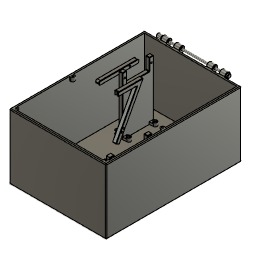
Useless_box (Autodesk Fusion 360 design; units mm, degrees)
Autodesk Fusion 360 part; units mm, degrees
note: some values were not read from the file. Set by a fixed rule: which face or edge a step refers to.
(part 1 of 2)
sketch "Sketch1" plane through (0, 0, 0) normal (0, 1, 0) x (1, 0, 0) in component "Box"
  line L0 (-60, -85) -> (60, -85)
  line L1 (60, -85) -> (60, 85)
  line L2 (60, 85) -> (-60, 85)
  line L3 (-60, 85) -> (-60, -85)
  line L4 (-60, -85) -> (60, 85) construction
  line L5 (60, -85) -> (-60, 85) construction
  dimension "d20" = 120
  dimension "d21" = 170
  constraint horizontal L0
  constraint perpendicular L0 L1
  constraint parallel L0 L2
  constraint parallel L1 L3
  constraint coincident L4 origin
  constraint coincident L5 origin
  measures "d20" distance of L1.end L2.end
  measures "d21" distance of L0.end L1.end
extrude "Extrude1" add sketch "Sketch1" along normal blind 3 makes body 1 in component "Box"
move_body "Move1" bodies 1 to x (1, 0, 0) y (0, 1, 0) z (0, 0, 1) at (0, 0, -10) in component "Box"
sketch "Sketch2" plane through (0, 3, 0) normal (0, 1, 0) x (-1, 0, 0) in component "Box"
  line L0 (60, -95) -> (60, 75)
  line L1 (60, 75) -> (-60, 75)
  line L2 (-60, 75) -> (-60, -95)
  line L3 (-60, -95) -> (60, -95)
  line L4 (60, -95) -> (60, -98)
  line L5 (60, -98) -> (63, -98)
  line L6 (63, -98) -> (63, 78)
  line L7 (63, 78) -> (-63, 78)
  line L8 (-63, 78) -> (-63, -98)
  line L9 (-63, -98) -> (63, -98)
  dimension "d26" = 3
  dimension "d27" = 3
  dimension "d28" = 176
  dimension "d29" = 126
  dimension "d30" = 176
  dimension "d31" = 126
  constraint coincident L0.start L3.end
  constraint perpendicular L3 L4
  constraint perpendicular L4 L5
  constraint perpendicular L5 L6
  constraint perpendicular L6 L7
  constraint perpendicular L7 L8
  constraint perpendicular L8 L9
  measures "d26" distance of L0.start L4.end
  measures "d27" distance of L4.end L5.end
  measures "d28" distance of L5.end L6.end
  measures "d29" distance of L6.end L7.end
  measures "d30" distance of L7.end L8.end
  measures "d31" distance of L8.end L5.end
extrude "Extrude2" add sketch "Sketch2" against normal up to surface (3 mm away) bodies 1 in component "Box"
sketch "Sketch3" plane through (0, 3, 0) normal (0, 1, 0) x (-1, 0, 0) in component "Box"
  line L0 (-63, -98) -> (63, -98)
  line L1 (63, -98) -> (63, 78)
  line L2 (63, 78) -> (-63, 78)
  line L3 (-63, 78) -> (-63, -98)
  line L4 (-60, -95) -> (60, -95)
  line L5 (60, -95) -> (60, 75)
  line L6 (60, 75) -> (-60, 75)
  line L7 (-60, 75) -> (-60, -95)
  line L8 (-60, -95) -> (60, 75) construction
  line L9 (60, -95) -> (-60, 75) construction
  line L10 (-14, -85) -> (-50, -85)
  line L11 (-50, -85) -> (-50, -29)
  line L12 (-50, -29) -> (-14, -29)
  line L13 (-14, -29) -> (-14, -85)
  circle A0 centre (-14, -85) radius 2.5
  circle A1 centre (-50, -85) radius 2.5
  circle A2 centre (-50, -29) radius 2.5
  circle A3 centre (-14, -29) radius 2.5
  circle A4 centre (-14, -85) radius 1.05
  circle A5 centre (-50, -85) radius 1.05
  circle A6 centre (-50, -29) radius 1.05
  circle A7 centre (-14, -29) radius 1.05
  line L14 (0, 0) -> (-22, 0)
  line L15 (-22, 0) -> (-22, -18)
  line L16 (-22, -18) -> (-27, -18)
  line L17 (-27, -18) -> (-27, 37)
  line L18 (-27, 37) -> (-22, 37)
  line L19 (-22, 37) -> (-22, 0)
  line L20 (39, -78) -> (34, -78)
  line L21 (39, -78) -> (39, -43.5)
  line L22 (34, -78) -> (34, -43.5)
  line L23 (34, -43.5) -> (39, -43.5)
  line L24 (39, -78) -> (39, -81)
  line L25 (39, -81) -> (34, -81)
  line L26 (34, -81) -> (34, -78)
  line L27 (39, -43.5) -> (39, -40.5)
  line L28 (39, -40.5) -> (34, -40.5)
  line L29 (34, -40.5) -> (34, -43.5)
  point P0 (0, -10)
  dimension "d34" = 120
  dimension "d35" = 170
  dimension "d36" = 36
  dimension "d37" = 56
  dimension "d38" = 10
  dimension "d39" = 10
  dimension "d40" = 5
  dimension "d41" = 5
  dimension "d42" = 5
  dimension "d43" = 5
  dimension "d44" = 2.1
  dimension "d45" = 2.1
  dimension "d46" = 2.1
  dimension "d47" = 2.1
  dimension "d50" = 22
  dimension "d51" = 18
  dimension "d52" = 5
  dimension "d53" = 55
  dimension "d54" = 5
  dimension "d76" = 5
  dimension "d77" = 17
  dimension "d78" = 34.5
  dimension "d79" = 21
  dimension "d80" = 3
  dimension "d81" = 5
  dimension "d82" = 3
  dimension "d83" = 5
  constraint horizontal L4
  constraint perpendicular L4 L5
  constraint parallel L4 L6
  constraint parallel L5 L7
  constraint coincident L8 P0
  constraint coincident L9 P0
  constraint horizontal L10
  constraint vertical L11
  constraint horizontal L12
  constraint vertical L13
  constraint coincident L10.start L13.end
  constraint coincident L10.end L11.start
  constraint coincident L11.end L12.start
  constraint coincident L12.end L13.start
  constraint concentric A0 A4
  constraint concentric A1 A5
  constraint concentric A2 A6
  constraint concentric A3 A7
  constraint coincident L14.start origin
  constraint horizontal L14
  constraint perpendicular L14 L15
  constraint perpendicular L15 L16
  constraint perpendicular L16 L17
  constraint perpendicular L17 L18
  constraint perpendicular L5 L20
  constraint perpendicular L20 L21
  constraint perpendicular L20 L22
  constraint perpendicular L21 L23
  constraint perpendicular L20 L24
  constraint perpendicular L24 L25
  constraint perpendicular L23 L27
  constraint perpendicular L27 L28
  measures "d34" distance of L5.end L6.end
  measures "d35" distance of L4.end L5.end
  measures "d36" distance of L10.start L10.end
  measures "d37" distance of L10.start L12.end
  measures "d38" distance of L7 L11
  measures "d39" distance of L4 L10
  measures "d40" diameter of A0
  measures "d41" diameter of A1
  measures "d42" diameter of A2
  measures "d43" diameter of A3
  measures "d44" diameter of A4
  measures "d45" diameter of A5
  measures "d46" diameter of A6
  measures "d47" diameter of A7
  measures "d50" distance of L14.start L14.end
  measures "d51" distance of L14.end L15.end
  measures "d52" distance of L15.end L16.end
  measures "d53" distance of L16.end L17.end
  measures "d54" distance of L17.end L18.end
  measures "d76" distance of L20.start L20.end
  measures "d77" distance of L4 L20
  measures "d78" distance of L20.start L21.end
  measures "d79" distance of L5 L21
  measures "d80" distance of L20.start L24.end
  measures "d81" distance of L24.end L25.end
  measures "d82" distance of L21.end L27.end
  measures "d83" distance of L27.end L28.end
extrude "Extrude9" add sketch "Sketch3" along normal blind 12 contours L10 L11 A1 A5 | L10 L11 A1 A5 | L10 L13 A0 A4 | L10 L13 A0 A4 | L11 L12 A2 A6 | L11 L12 A2 A6 | L12 L13 A3 A7 | L12 L13 A3 A7 bodies 1 in component "Box"
sketch "Sketch1 (2)" plane through (0, 3, 0) normal (0, 1, 0) x (-1, 0, 0) in component "Switch_servo_mount"
  circle A0 centre (-50, -29) radius 2.5
  circle A1 centre (-14, -29) radius 2.5
  line L0 (-63, -98) -> (63, -98)
  line L1 (63, -98) -> (63, 78)
  line L2 (63, 78) -> (-63, 78)
  line L3 (-63, 78) -> (-63, -98)
  circle A2 centre (-14, -85) radius 2.5
  circle A3 centre (-50, -85) radius 2.5
  line L4 (-22, -18) -> (-27, -18)
  line L5 (-27, -18) -> (-27, 37)
  line L6 (-27, 37) -> (-22, 37)
  line L7 (-22, 37) -> (-22, -18)
  line L8 (0, 0) -> (-22, 0) construction
  line L9 (-22, -18) -> (-17, -18)
  circle A4 centre (-17, -15) radius 2.5
  circle A5 centre (-32, -15) radius 2.5
  line L10 (-22, -18) -> (-27, -18)
  circle A6 centre (-17, 34) radius 2.5
  circle A7 centre (-32, 34) radius 2.5
  line L11 (-27, 37) -> (-22, 37)
  line L12 (-22, 37) -> (-16.7571, 36.4882)
  line L13 (-27, 37) -> (-32.2429, 36.4882)
  line L14 (-32.2429, 31.5118) -> (-27, 31)
  line L15 (-17, 31.5) -> (-22, 31)
  line L16 (-22, -18) -> (-16.7571, -17.4882)
  line L17 (-16.7571, -12.5118) -> (-22, -12)
  line L18 (-27, -18) -> (-32.2429, -17.4882)
  line L19 (-32, -12.5) -> (-27, -11.7993)
  circle A8 centre (-17, -15) radius 1.05
  circle A9 centre (-32, -15) radius 1.05
  circle A10 centre (-17, 34) radius 1.05
  circle A11 centre (-32, 34) radius 1.05
  line L20 (39, -40.5) -> (39, -81)
  line L21 (39, -81) -> (34, -81)
  line L22 (34, -81) -> (34, -40.5)
  line L23 (34, -40.5) -> (39, -40.5)
  circle A12 centre (44, -78) radius 2.5
  circle A13 centre (29, -78) radius 2.5
  circle A14 centre (44, -43.5) radius 2.5
  circle A15 centre (29, -43.5) radius 2.5
  line L24 (39, -40.5) -> (34, -40.5)
  line L25 (34, -81) -> (28.7571, -80.4882)
  line L26 (39, -81) -> (44.2429, -80.4882)
  line L27 (44, -75.5) -> (39, -75.0119)
  line L28 (29, -75.5) -> (34, -75.0119)
  line L29 (39, -40.5) -> (44.2429, -41.0118)
  line L30 (34, -40.5) -> (28.7571, -41.0118)
  line L31 (28.7571, -45.9882) -> (34, -46.5)
  line L32 (39, -46.5) -> (44.2429, -45.9882)
  point P0 (34, -78)
  point P1 (39, -78)
  point P2 (39, -43.5)
  point P3 (34, -43.5)
  dimension "d118" = 5
  dimension "d119" = 5
  dimension "d120" = 5
  dimension "d121" = 3
  dimension "d122" = 5
  dimension "d123" = 3
  dimension "d124" = 5
  dimension "d125" = 5
  dimension "d126" = 5
  dimension "d127" = 3
  dimension "d128" = 3
  dimension "d129" = 5
  dimension "d130" = 5
  dimension "d131" = 2.1
  dimension "d132" = 2.1
  dimension "d133" = 2.1
  dimension "d134" = 2.1
  dimension "d193" = 5
  dimension "d196" = 5
  dimension "d197" = 5
  dimension "d198" = 5
  dimension "d199" = 5
  dimension "d200" = 5
  dimension "d201" = 5
  dimension "d202" = 5
  dimension "d203" = 5
  dimension "d204" = 3
  dimension "d205" = 3
  dimension "d206" = 3
  dimension "d207" = 3
  constraint horizontal L4
  constraint perpendicular L4 L5
  constraint perpendicular L5 L6
  constraint perpendicular L4 L7
  constraint coincident L8.start origin
  constraint coincident L7 L8.end
  constraint perpendicular L7 L8
  constraint perpendicular L7 L9
  constraint coincident L6.end L7.start
  constraint coincident A6 L12.end
  constraint tangent A6 L12
  constraint coincident L5.end L6.start
  constraint coincident A7 L13.end
  constraint tangent A7 L13
  constraint coincident A7 L14.start
  constraint coincident L5 L14.end
  constraint tangent A7 L14
  constraint coincident A6 L15.start
  constraint coincident L7 L15.end
  constraint coincident L4.start L7.end
  constraint coincident A4 L16.end
  constraint tangent A4 L16
  constraint coincident A4 L17.start
  constraint coincident L7 L17.end
  constraint tangent A4 L17
  constraint coincident L4.end L5.start
  constraint coincident A5 L18.end
  constraint tangent A5 L18
  constraint coincident A5 L19.start
  constraint coincident L5 L19.end
  constraint concentric A4 A8
  constraint concentric A5 A9
  constraint concentric A6 A10
  constraint concentric A7 A11
  constraint vertical L20
  constraint perpendicular L20 L21
  constraint perpendicular L21 L22
  constraint perpendicular L20 L23
  constraint coincident A13 L25.end
  constraint tangent A13 L25
  constraint coincident A12 L26.end
  constraint tangent A12 L26
  constraint coincident A12 L27.start
  constraint coincident L20 L27.end
  constraint parallel L25 L27
  constraint coincident A13 L28.start
  constraint coincident L22 L28.end
  constraint parallel L26 L28
  constraint coincident A14 L29.end
  constraint tangent A14 L29
  constraint coincident L22.end L23.start
  constraint coincident A15 L30.end
  constraint tangent A15 L30
  constraint coincident A15 L31.start
  constraint coincident L22 L31.end
  constraint tangent A15 L31
  constraint coincident L20 L32.start
  constraint coincident A14 L32.end
  constraint tangent A14 L32
  measures "d118" distance of L4.start L9.end
  measures "d119" diameter of A4
  measures "d120" diameter of A5
  measures "d121" distance of L9 A4.centre
  measures "d122" distance of L7 A4.centre
  measures "d123" distance of A5.centre L10
  measures "d124" distance of L5 A5.centre
  measures "d125" diameter of A6
  measures "d126" diameter of A7
  measures "d127" distance of A7.centre L11
  measures "d128" distance of L6 A6.centre
  measures "d129" distance of L7 A6.centre
  measures "d130" distance of L5 A7.centre
  measures "d131" diameter of A8
  measures "d132" diameter of A9
  measures "d133" diameter of A10
  measures "d134" diameter of A11
  measures "d193" distance of L20.end L21.end
  measures "d196" diameter of A12
  measures "d197" diameter of A13
  measures "d198" diameter of A14
  measures "d199" diameter of A15
  measures "d200" distance of A13.centre P0
  measures "d201" distance of A12.centre P1
  measures "d202" distance of A14.centre P2
  measures "d203" horizontal distance of A15.centre P3
  measures "d204" distance of L23 A15.centre
  measures "d205" distance of A14.centre L24
  measures "d206" distance of L21 A12.centre
  measures "d207" distance of L21 A13.centre
sketch "Sketch1 (3)" plane through (0, 3, 0) normal (0, 1, 0) x (-1, 0, 0) in component "Lid_servo_mount"
  circle A0 centre (-50, -29) radius 2.5
  circle A1 centre (-14, -29) radius 2.5
  line L0 (-63, -98) -> (63, -98)
  line L1 (63, -98) -> (63, 78)
  line L2 (63, 78) -> (-63, 78)
  line L3 (-63, 78) -> (-63, -98)
  circle A2 centre (-14, -85) radius 2.5
  circle A3 centre (-50, -85) radius 2.5
  line L4 (34, -40.5) -> (39, -40.5)
  line L5 (39, -40.5) -> (39, -81)
  line L6 (39, -81) -> (34, -81)
  line L7 (34, -81) -> (34, -40.5)
  circle A4 centre (44, -78) radius 2.5
  circle A5 centre (29, -78) radius 2.5
  circle A6 centre (44, -43.5) radius 2.5
  circle A7 centre (29, -43.5) radius 2.5
  line L8 (39, -40.5) -> (44.2429, -41.0118)
  line L9 (44.2429, -45.9882) -> (39, -46.5)
  line L10 (34, -40.5) -> (28.7571, -41.0118)
  line L11 (28.7571, -45.9882) -> (34, -46.5)
  line L12 (39, -81) -> (44.2429, -80.4882)
  line L13 (34, -81) -> (28.7571, -80.4882)
  line L14 (28.7571, -75.5118) -> (34, -75)
  line L15 (39, -75) -> (44.2429, -75.5118)
  circle A8 centre (44, -78) radius 1.05
  circle A9 centre (29, -78) radius 1.05
  circle A10 centre (29, -43.5) radius 1.05
  circle A11 centre (44, -43.5) radius 1.05
  dimension "d208" = 5
  dimension "d209" = 5
  dimension "d210" = 5
  dimension "d211" = 5
  dimension "d212" = 5
  dimension "d213" = 5
  dimension "d214" = 2.1
  dimension "d215" = 2.1
  dimension "d216" = 2.1
  dimension "d217" = 2.1
  constraint horizontal L4
  constraint perpendicular L4 L5
  constraint perpendicular L5 L6
  constraint coincident A6 L8.end
  constraint tangent A6 L8
  constraint coincident A6 L9.start
  constraint coincident L5 L9.end
  constraint tangent A6 L9
  constraint coincident A7 L10.end
  constraint tangent A7 L10
  constraint coincident A7 L11.start
  constraint coincident L7 L11.end
  constraint tangent A7 L11
  constraint coincident A4 L12.end
  constraint tangent A4 L12
  constraint coincident A5 L13.end
  constraint tangent A5 L13
  constraint coincident A5 L14.start
  constraint coincident L7 L14.end
  constraint tangent A5 L14
  constraint coincident L5 L15.start
  constraint coincident A4 L15.end
  constraint tangent A4 L15
  constraint concentric A4 A8
  constraint concentric A5 A9
  constraint concentric A7 A10
  constraint concentric A6 A11
  measures "d208" distance of L4.start L4.end
  measures "d209" distance of L5.end L6.end
  measures "d210" diameter of A4
  measures "d211" diameter of A5
  measures "d212" diameter of A6
  measures "d213" diameter of A7
  measures "d214" diameter of A8
  measures "d215" diameter of A9
  measures "d216" diameter of A10
  measures "d217" diameter of A11
extrude "Extrude1'" add sketch "Sketch1 (3)" along normal blind 3 separate body contours L5 A6 L8 L9 makes body 2 in component "Lid_servo_mount"
extrude "Extrude2'" add sketch "Sketch1 (2)" along normal blind 75 contours L20 L21 L22 L23 L24 bodies 2 in component "Lid_servo_mount"
extrude "Extrude3" add sketch "Sketch1 (2)" along normal blind 3 contours L22 A15 L30 L31 | L20 A12 L26 L27 | L22 A13 L25 L28 bodies 2 in component "Lid_servo_mount"
extrude "Extrude4" add sketch "Sketch1 (3)" along normal blind 5 contours A7 | A6 | A5 | A4 bodies 2 in component "Lid_servo_mount"
extrude "Extrude1''" add sketch "Sketch1 (2)" along normal blind 49 separate body contours L4 L5 L6 L7 L10 L11 makes body 3 in component "Switch_servo_mount"
extrude "Extrude2''" add sketch "Sketch1 (2)" along normal blind 3 contours L7 A4 L16 L17 | L5 A5 L18 L19 | L7 A6 L12 L15 | L5 A7 L13 L14 bodies 3 in component "Switch_servo_mount"
extrude "Extrude3'" add sketch "Sketch1 (2)" along normal blind 5 contours A4 | A5 | A6 | A7 bodies 3 in component "Switch_servo_mount"
sketch "Sketch2 (2)" plane through (22, 0, 0) normal (-1, 0, 0) x (0, 0, 1) in component "Switch_servo_mount"
  line L0 (-12, 6) -> (-12, 3)
  line L1 (-12, 3) -> (31, 3)
  line L2 (31, 3) -> (31, 6)
  line L3 (31, 6) -> (37, 6)
  line L4 (37, 6) -> (37, 52)
  line L5 (37, 52) -> (-18, 52)
  line L6 (-18, 52) -> (-18, 6)
  line L7 (-18, 6) -> (-12, 6)
  line L8 (-15, 52) -> (-15, 32) construction
  line L9 (34, 52) -> (34, 32) construction
  line L10 (31, 52) -> (31, 32) construction
  line L11 (-12, 52) -> (-12, 32) construction
  circle A0 centre (-15, 45) radius 0.85
  circle A1 centre (-15, 39) radius 0.85
  circle A2 centre (34, 45) radius 0.85
  line L12 (-15, 42) -> (34, 42) construction
  circle A3 centre (34, 39) radius 0.85
  line L13 (-12, 32) -> (31, 32)
  line L14 (31, 52) -> (31, 32)
  line L15 (31, 52) -> (-12, 52)
  line L16 (-12, 52) -> (-12, 32)
  circle A4 centre (0, 42) radius 2.5
  dimension "d141" = 20
  dimension "d142" = 20
  dimension "d143" = 3
  dimension "d144" = 3
  dimension "d145" = 20
  dimension "d147" = 20
  dimension "d148" = 3
  dimension "d149" = 3
  dimension "d150" = 1.7
  dimension "d151" = 1.7
  dimension "d152" = 1.7
  dimension "d153" = 1.7
  dimension "d154" = 3
  dimension "d155" = 3
  dimension "d156" = 3
  dimension "d157" = 3
  dimension "d158" = 5
  dimension "d159" = 10
  dimension "d161" = 15
  constraint coincident L5 L8.start
  constraint perpendicular L5 L8
  constraint coincident L5 L9.start
  constraint perpendicular L5 L9
  constraint coincident L5 L10.start
  constraint perpendicular L5 L10
  constraint coincident L5 L11.start
  constraint perpendicular L5 L11
  constraint coincident L8 A0.centre
  constraint coincident L8 A1.centre
  constraint coincident L9 A2.centre
  constraint midpoint L8 L12.start
  constraint midpoint L9 L12.end
  constraint coincident L9 A3.centre
  measures "d141" distance of L8.start L8.end
  measures "d142" distance of L9.start L9.end
  measures "d143" distance of L6 L8
  measures "d144" distance of L4 L9
  measures "d145" distance of L10.start L10.end
  measures "d147" distance of L11.start L11.end
  measures "d148" distance of L9 L10
  measures "d149" distance of L8 L11
  measures "d150" diameter of A0
  measures "d151" diameter of A1
  measures "d152" diameter of A2
  measures "d153" diameter of A3
  measures "d154" distance of A0.centre L12.start
  measures "d155" distance of A1.centre L12.start
  measures "d156" distance of L12.end A3.centre
  measures "d157" distance of A2.centre L12.end
  measures "d158" diameter of A4
  measures "d159" distance of L15 A4.centre
  measures "d161" distance of L12.start A4.centre
extrude "Extrude4'" cut sketch "Sketch2 (2)" against normal blind 5 contours L5 L13 L14 L15 L16 | A0 | A1 | A2 | A3 | A4 bodies 3 in component "Switch_servo_mount"
sketch "Sketch2 (3)" plane through (-39, 0, 0) normal (-1, 0, 0) x (0, 0, 1) in component "Lid_servo_mount"
  line L0 (-75.0119, 6) -> (-75.0119, 3)
  line L1 (-75.0119, 3) -> (-46.5, 3)
  line L2 (-46.5, 3) -> (-46.5, 6)
  line L3 (-46.5, 6) -> (-40.5, 6)
  line L4 (-40.5, 6) -> (-40.5, 78)
  line L5 (-40.5, 78) -> (-81, 78)
  line L6 (-81, 78) -> (-81, 6)
  line L7 (-81, 6) -> (-75.0119, 6)
  line L8 (-78, 78) -> (-78, 64.5) construction
  line L9 (-78, 64.5) -> (-43.5, 64.5)
  line L10 (-43.5, 64.5) -> (-40.5, 64.5)
  line L11 (-43.5, 64.5) -> (-43.5, 78) construction
  line L12 (-78, 71.25) -> (-43.5, 71.25) construction
  line L13 (-46, 78) -> (-46, 64.5)
  line L14 (-75.5, 78) -> (-75.5, 64.5)
  circle A0 centre (-78, 71.25) radius 1
  circle A1 centre (-43.5, 71.25) radius 1
  dimension "d226" = 13.5
  dimension "d227" = 3
  dimension "d228" = 34.5
  dimension "d229" = 3
  dimension "d230" = 2.5
  dimension "d231" = 2.5
  dimension "d232" = 2
  dimension "d233" = 2
  constraint coincident L5 L8.start
  constraint perpendicular L5 L8
  constraint perpendicular L8 L9
  constraint perpendicular L4 L10
  constraint coincident L5 L11.end
  constraint perpendicular L5 L11
  constraint midpoint L8 L12.start
  constraint midpoint L11 L12.end
  constraint coincident L5 L13.start
  constraint coincident L9 L13.end
  constraint perpendicular L9 L13
  constraint coincident L5 L14.start
  constraint coincident L9 L14.end
  constraint perpendicular L9 L14
  constraint coincident L12.start A0.centre
  constraint coincident L12.end A1.centre
  measures "d226" distance of L8.start L8.end
  measures "d227" distance of L6 L8
  measures "d228" distance of L8.end L9.end
  measures "d229" distance of L9.end L10.end
  measures "d230" distance of L8 L14
  measures "d231" distance of L11 L13
  measures "d232" diameter of A0
  measures "d233" diameter of A1
extrude "Extrude5" cut sketch "Sketch2 (3)" against normal blind 5 contours L5 L9 L13 L14 | A0 | A1 bodies 2 in component "Lid_servo_mount"
move_face "OffsetFaces1" offset -2 1 faces at (-35.6667, 64.5, -65.6667) on bodies 2 in component "Lid_servo_mount"
move_face "OffsetFaces1'" offset -2 1 faces at (23.6667, 32, 2.3333) on bodies 3 in component "Switch_servo_mount"
move_face "OffsetFaces4" offset 2 1 faces at (-21, 0, -39.3333) on bodies 1 in component "Box"
sketch "Sketch7" plane through (0, 3, 0) normal (0, 1, 0) x (-1, 0, 0) in component "Box"
  circle A0 centre (-50, -29) radius 2.5
  circle A1 centre (-14, -29) radius 2.5
  line L0 (-63, -98) -> (63, -98)
  line L1 (63, -98) -> (63, 78)
  line L2 (63, 78) -> (-63, 78)
  line L3 (-63, 78) -> (-63, -98)
  circle A2 centre (-14, -85) radius 2.5
  circle A3 centre (-50, -85) radius 2.5
  circle A4 centre (44, -78) radius 1.05
  circle A5 centre (29, -78) radius 1.05
  circle A6 centre (44, -43.5) radius 1.05
  circle A7 centre (29, -43.5) radius 1.05
  circle A8 centre (-17, -15) radius 1.05
  circle A9 centre (-32, -15) radius 1.05
  circle A10 centre (-17, 34) radius 1.05
  circle A11 centre (-32, 34) radius 1.05
  dimension "d239" = 2.1
  dimension "d240" = 2.1
  dimension "d241" = 2.1
  dimension "d242" = 2.1
  dimension "d243" = 2.1
  dimension "d244" = 2.1
  dimension "d245" = 2.1
  dimension "d246" = 2.1
  measures "d239" diameter of A4
  measures "d240" diameter of A5
  measures "d241" diameter of A6
  measures "d242" diameter of A7
  measures "d243" diameter of A8
  measures "d244" diameter of A9
  measures "d245" diameter of A10
  measures "d246" diameter of A11
extrude "Extrude10" cut sketch "Sketch7" against normal blind 5 contours A4 | A5 | A6 | A7 | A8 | A9 | A10 | A11 bodies 1 in component "Box"
sketch "Sketch1 (4)" plane through (0, 0, 0) normal (1, 0, 0) x (0, 0, -1) in component "Finger_switch"
  line L0 (0, 0) -> (0, 97) construction
  line L1 (-75, 0) -> (-75, 83) construction
  line L2 (-78, 0) -> (10, 0) construction
  line L3 (10, 0) -> (10, 83) construction
  line L4 (0, 42) -> (25.8241, 90.5605)
  line L5 (-2.1759, 90.5605) -> (-2.1759, 95.5605)
  line L6 (0, 42) -> (-2.2073, 43.1738)
  line L7 (0, 42) -> (2.2073, 40.8262)
  line L8 (-2.2073, 43.1738) -> (22.9925, 90.5605)
  line L9 (22.9925, 90.5605) -> (-2.1759, 90.5605)
  line L10 (-2.1759, 95.5605) -> (28.483, 95.5605)
  line L11 (28.483, 95.5605) -> (25.8241, 90.5605)
  line L12 (2.2073, 40.8262) -> (31.3145, 95.5605)
  line L13 (31.3145, 95.5605) -> (28.483, 95.5605)
  line L14 (-2.1759, 93.0605) -> (27.1535, 93.0605)
  line L15 (2.2073, 40.8262) -> (-0.1403, 36.4116)
  line L16 (-0.1403, 36.4116) -> (-4.5549, 38.7592)
  line L17 (-4.5549, 38.7592) -> (-2.2073, 43.1738)
  dimension "d164" = 97
  dimension "d165" = 83
  dimension "d166" = 88
  dimension "d167" = 83
  dimension "d168" = 55
  dimension "d169" = 28
  dimension "d170" = 5
  dimension "d171" = 2.5
  dimension "d172" = 2.5
  dimension "d173" = 5
  dimension "d174" = 5
  dimension "d175" = 5
  constraint coincident L0.start origin
  constraint vertical L0
  constraint vertical L1
  constraint perpendicular L1 L2
  constraint perpendicular L2 L3
  constraint coincident L0 L4.start
  constraint perpendicular L4 L6
  constraint perpendicular L4 L7
  constraint perpendicular L6 L8
  constraint perpendicular L5 L9
  constraint perpendicular L5 L10
  constraint parallel L4 L11
  constraint perpendicular L7 L12
  constraint parallel L10 L13
  constraint midpoint L5 L14.start
  constraint midpoint L11 L14.end
  constraint perpendicular L5 L14
  constraint perpendicular L7 L15
  constraint perpendicular L15 L16
  constraint perpendicular L6 L17
  measures "d164" distance of L0.start L0.end
  measures "d165" distance of L1.start L1.end
  measures "d166" distance of L2.start L2.end
  measures "d167" distance of L2.end L3.end
  measures "d168" distance of L4.start L4.end
  measures "d169" distance of L4.end L5.start
  measures "d170" distance of L5.start L5.end
  measures "d171" distance of L4.start L6.end
  measures "d172" distance of L4.start L7.end
  measures "d173" distance of L7.end L15.end
  measures "d174" distance of L15.end L16.end
  measures "d175" distance of L16.end L6.end
extrude "Extrude1'''" add sketch "Sketch1 (4)" along normal mid plane 5 separate body makes body 4 in component "Finger_switch"
sketch "Sketch2 (4)" plane through (0, 95.5605, 0) normal (0, 1, 0) x (-1, 0, 0) in component "Finger_switch"
  line L0 (2.5, 2.1759) -> (-2.5, 2.1759)
  line L1 (-2.5, 2.1759) -> (-2.5, -31.3145)
  line L2 (-2.5, -31.3145) -> (2.5, -31.3145)
  line L3 (2.5, -31.3145) -> (2.5, 2.1759)
  line L4 (0, 2.1759) -> (0, -0.8241)
  line L5 (-2.5, 2.1759) -> (0, -0.8241)
  line L6 (2.5, 2.1759) -> (0, -0.8241)
  line L7 (0, 2.1759) -> (0, 0.1759)
  line L8 (-2.5, 2.1759) -> (0, 0.1759)
  line L9 (0, 0.1759) -> (2.5, 2.1759)
  dimension "d178" = 3
  dimension "d187" = 2
  constraint midpoint L0 L4.start
  constraint perpendicular L0 L4
  constraint coincident L0.end L1.start
  constraint coincident L0.start L3.end
  constraint perpendicular L0 L7
  measures "d178" distance of L4.start L4.end
  measures "d187" distance of L4.start L7.end
extrude "Extrude4''" cut sketch "Sketch2 (4)" against normal up to surface (5 mm away) contours L0 L4 L7 L9 | L0 L4 L7 L8 bodies 4 in component "Finger_switch"
extrude "Extrude2'''" cut sketch "Sketch2 (4)" against normal up to surface (5 mm away) contours L0 L4 L7 L9 | L4 L6 L9 | L0 L4 L7 L8 | L4 L5 L8 bodies 4 in component "Finger_switch"
sketch "Sketch3 (2)" plane through (-2.5, 0, 0) normal (-1, 0, 0) x (0, 0, 1) in component "Finger_switch"
  line L0 (-31.3145, 95.5605) -> (0.1403, 36.4116)
  line L1 (0.1403, 36.4116) -> (4.5549, 38.7592)
  line L2 (4.5549, 38.7592) -> (-22.9925, 90.5605)
  line L3 (-22.9925, 90.5605) -> (2.1759, 90.5605)
  line L4 (2.1759, 90.5605) -> (2.1759, 95.5605)
  line L5 (2.1759, 95.5605) -> (-31.3145, 95.5605)
  line L6 (0, 42) -> (-3.2867, 48.1804)
  circle A0 centre (-3.2867, 48.1804) radius 1.05
  line L7 (0, 42) -> (-5.1648, 51.7121)
  circle A1 centre (-5.1648, 51.7121) radius 1.05
  dimension "d181" = 7
  dimension "d182" = 2.1
  dimension "d183" = 11
  dimension "d184" = 2.1
  constraint parallel L2 L6
  constraint coincident L6.end A0.centre
  constraint parallel L6 L7
  constraint coincident L7.end A1.centre
  measures "d181" distance of L6.start L6.end
  measures "d182" diameter of A0
  measures "d183" distance of L6.start L7.end
  measures "d184" diameter of A1
extrude "Extrude3''" cut sketch "Sketch3 (2)" against normal up to surface (5 mm away) contours L6 A0 L7 | L6 A0 L7 | A1 bodies 4 in component "Finger_switch"
extrude "Extrude5'" add sketch "Sketch2 (4)" against normal up to surface (5 mm away) contours L4 L6 L9 | L4 L5 L8 bodies 4 in component "Finger_switch"
fillet "Fillet1" radius 0.5 21 edges at (-2.5, 93.0605, 2.1759) (2.5, 93.0605, 2.1759) (-1.25, 90.5605, 1.1759) (1.25, 90.5605, 1.1759) (-1.25, 95.5605, 1.1759) (1.25, 95.5605, 1.1759) (0, 93.0605, 0.1759) (-2.5, 95.5605, -14.5693) (2.5, 95.5605, -14.5693) (0, 95.5605, -31.3145) (-2.5, 90.5605, -10.4083) (-2.5, 64.6598, -9.2188) (-2.5, 65.986, -15.5871) (0, 90.5605, -22.9925) (2.5, 90.5605, -10.4083) (2.5, 64.6598, -9.2188) (2.5, 65.986, -15.5871) (0, 36.4116, 0.1403) (-2.5, 37.5854, 2.3476) (0, 38.7592, 4.5549) (2.5, 37.5854, 2.3476) on bodies 4 in component "Finger_switch"
sketch "Sketch1 (5)" plane through (-39, 0, 0) normal (-1, 0, 0) x (0, 0, 1) in component "Finger_lid"
  line L0 (-46, 78) -> (-46, 62.5)
  line L1 (-46, 62.5) -> (-75.5, 62.5)
  line L2 (-75.5, 62.5) -> (-75.5, 78)
  line L3 (-75.5, 78) -> (-81, 78)
  line L4 (-81, 78) -> (-81, 6)
  line L5 (-81, 6) -> (-75.0119, 6)
  line L6 (-75.0119, 6) -> (-75.0119, 3)
  line L7 (-75.0119, 3) -> (-46.5, 3)
  line L8 (-46.5, 3) -> (-46.5, 6)
  line L9 (-46.5, 6) -> (-40.5, 6)
  line L10 (-40.5, 6) -> (-40.5, 78)
  line L11 (-40.5, 78) -> (-46, 78)
  circle A0 centre (-43.5, 71.25) radius 1
  circle A1 centre (-78, 71.25) radius 1
  line L12 (-78, 71.25) -> (-67, 71.25) construction
  circle A2 centre (-67, 71.25) radius 2.5 construction
  line L13 (-13.5581, 3) -> (-13.5581, 83) construction
  line L14 (-67, 71.25) -> (-20, 71.25) construction
  line L15 (-67, 71.25) -> (-67, 73.75)
  line L16 (-67, 71.25) -> (-67, 68.75)
  line L17 (-67, 73.75) -> (-72, 73.75)
  line L18 (-72, 73.75) -> (-72, 68.75)
  line L19 (-72, 68.75) -> (-20, 68.75)
  line L20 (-20, 68.75) -> (-20, 73.75)
  line L21 (-20, 73.75) -> (-67, 73.75)
  dimension "d249" = 11
  dimension "d250" = 5
  dimension "d251" = 80
  dimension "d252" = 47
  dimension "d253" = 2.5
  dimension "d254" = 2.5
  dimension "d255" = 5
  dimension "d256" = 5
  dimension "d257" = 5
  constraint coincident A1.centre L12.start
  constraint perpendicular L2 L12
  constraint coincident L12.end A2.centre
  constraint perpendicular L7 L13
  constraint perpendicular L13 L14
  constraint perpendicular L12 L15
  constraint perpendicular L12 L16
  constraint perpendicular L15 L17
  constraint perpendicular L12 L18
  constraint perpendicular L18 L19
  constraint perpendicular L14 L20
  measures "d249" distance of A1.centre L12.end
  measures "d250" diameter of A2
  measures "d251" distance of L13.start L13.end
  measures "d252" distance of L12.end L14.end
  measures "d253" distance of L12.end L15.end
  measures "d254" distance of L12.end L16.end
  measures "d255" distance of L15.end L17.end
  measures "d256" distance of L17.end L18.end
  measures "d257" distance of L19.end L20.end
extrude "Extrude1''''" add sketch "Sketch1 (5)" along normal blind 5 separate body contours L0 L10 L19 L21 | L0 L15 L16 L19 L21 | L10 L19 L20 L21 | L15 L16 L17 L18 L19 | A0 makes body 5 in component "Finger_lid"
move_body "Move1'" bodies 5 to x (1, 0, 0) y (0, 1, 0) z (0, 0, 1) at (-5, 0, 0) in component "Finger_lid"
sketch "Sketch2 (5)" plane through (-49, 0, 0) normal (-1, 0, 0) x (0, 0, 1) in component "Finger_lid"
  line L0 (-20, 73.75) -> (-72, 73.75)
  line L1 (-72, 73.75) -> (-72, 68.75)
  line L2 (-72, 68.75) -> (-20, 68.75)
  line L3 (-20, 68.75) -> (-20, 73.75)
  line L4 (-72, 71.25) -> (-67, 71.25)
  line L5 (-67, 71.25) -> (-60, 71.25)
  circle A0 centre (-60, 71.25) radius 1.05
  line L6 (-60, 71.25) -> (-51, 71.25)
  circle A1 centre (-51, 71.25) radius 1.05
  dimension "d260" = 7
  dimension "d261" = 2.1
  dimension "d262" = 9
  dimension "d263" = 2.1
  constraint midpoint L1 L4.start
  constraint perpendicular L1 L4
  constraint parallel L4 L5
  constraint coincident L5.end A0.centre
  constraint parallel L5 L6
  constraint coincident L6.end A1.centre
  measures "d260" distance of L4.end L5.end
  measures "d261" diameter of A0
  measures "d262" distance of L5.end L6.end
  measures "d263" diameter of A1
extrude "Extrude2''''" cut sketch "Sketch2 (5)" against normal up to surface (5 mm away) contours L5 A0 L6 | L5 A0 L6 | A1 bodies 5 in component "Finger_lid"
fillet "Fillet1'" radius 0.5 8 edges at (-49, 73.75, -46) (-49, 68.75, -46) (-49, 71.25, -20) (-44, 71.25, -20) (-44, 73.75, -46) (-49, 71.25, -72) (-44, 71.25, -72) (-44, 68.75, -46) on bodies 5 in component "Finger_lid"
fillet "Fillet2" radius 2 12 edges at (-44.1464, 73.6036, -20.1464) (-46.5, 73.75, -20) (-48.8536, 73.6036, -20.1464) (-44.1464, 68.8964, -20.1464) (-46.5, 68.75, -20) (-48.8536, 68.8964, -20.1464) (-44.1464, 73.6036, -71.8536) (-46.5, 73.75, -72) (-48.8536, 73.6036, -71.8536) (-44.1464, 68.8964, -71.8536) (-46.5, 68.75, -72) (-48.8536, 68.8964, -71.8536) on bodies 5 in component "Finger_lid"
extrude "Extrude11" add sketch "Sketch2" along normal blind 80 bodies 1 in component "Box"
sketch "Sketch3 (3)" plane through (0, 83, 0) normal (0, 1, 0) x (-1, 0, 0) in component "Lid"
  line L0 (60, -95) -> (-60, -95)
  line L1 (-60, -95) -> (-60, 75)
  line L2 (-60, 75) -> (60, 75)
  line L3 (60, 75) -> (60, -95)
  line L4 (-63, -98) -> (63, -98)
  line L5 (63, -98) -> (63, 78)
  line L6 (63, 78) -> (-63, 78)
  line L7 (-63, 78) -> (-63, -98)
  line L8 (63, 78) -> (-63, 78)
  line L9 (-63, 78) -> (-63, -10)
  line L10 (-63, -10) -> (63, -10)
  line L11 (63, -10) -> (63, 78)
  dimension "d270" = 126
  dimension "d271" = 88
  constraint horizontal L8
  constraint vertical L9
  constraint horizontal L10
  constraint vertical L11
  constraint coincident L5.end L6.start
  measures "d270" distance of L5.end L6.end
  measures "d271" distance of L5.end L10.end
extrude "Extrude3'''" add sketch "Sketch3 (3)" along normal blind 3 separate body contours L1 L2 L3 L10 | L1 L2 L3 L5 L6 L7 L8 L9 L10 L11 makes body 6 in component "Lid"
sketch "Sketch4" plane through (0, 86, 0) normal (0, 1, 0) x (-1, 0, 0) in component "Lid"
  line L0 (63, -10) -> (63, 78)
  line L1 (63, 78) -> (-63, 78)
  line L2 (-63, 78) -> (-63, -10)
  line L3 (-63, -10) -> (63, -10)
  circle A0 centre (0, 0) radius 3.1
  dimension "d274" = 6.2
  constraint coincident A0.centre origin
  measures "d274" diameter of A0
extrude "Extrude4'''" cut sketch "Sketch4" against normal up to surface (3 mm away) contours A0 bodies 6 in component "Lid"
sketch "Sketch5" plane through (0, 86, 0) normal (0, 1, 0) x (-1, 0, 0) in component "Lid"
  circle A0 centre (0, 0) radius 3.1
  line L0 (63, -10) -> (63, 78)
  line L1 (63, 78) -> (-63, 78)
  line L2 (-63, 78) -> (-63, -10)
  line L3 (-63, -10) -> (63, -10)
  circle A1 centre (58.5, 0) radius 3
  circle A2 centre (-58.5, 0) radius 3
  circle A3 centre (58.5, 73.5) radius 3
  circle A4 centre (-58.5, 73.5) radius 3
  line L4 (58.5, 70.5) -> (63, 70.5)
  line L5 (55.5, 73.5) -> (55.5, 78)
  line L6 (-55.5, 73.5) -> (-55.5, 78)
  line L7 (-58.5, 70.5) -> (-63, 70.5)
  line L8 (-58.5, -3) -> (-63, -3)
  line L9 (-58.5, 3) -> (-63, 3)
  line L10 (58.5, -3) -> (63, -3)
  line L11 (58.5, 3) -> (63, 3)
  circle A5 centre (-58.5, 0) radius 1.05
  circle A6 centre (-58.5, 73.5) radius 1.05
  circle A7 centre (58.5, 73.5) radius 1.05
  circle A8 centre (58.5, 0) radius 1.05
  dimension "d298" = 6
  dimension "d299" = 6
  dimension "d300" = 4.5
  dimension "d301" = 4.5
  dimension "d302" = 6
  dimension "d303" = 6
  dimension "d304" = 4.5
  dimension "d305" = 4.5
  dimension "d306" = 4.5
  dimension "d307" = 4.5
  dimension "d308" = 2.1
  dimension "d309" = 2.1
  dimension "d310" = 2.1
  dimension "d311" = 2.1
  constraint coincident A3 L4.start
  constraint coincident L0 L4.end
  constraint tangent A3 L4
  constraint perpendicular L0 L4
  constraint coincident A3 L5.start
  constraint coincident L1 L5.end
  constraint tangent A3 L5
  constraint perpendicular L1 L5
  constraint coincident A4 L6.start
  constraint coincident L1 L6.end
  constraint tangent A4 L6
  constraint perpendicular L1 L6
  constraint coincident A4 L7.start
  constraint coincident L2 L7.end
  constraint tangent A4 L7
  constraint perpendicular L2 L7
  constraint coincident A2 L8.start
  constraint coincident L2 L8.end
  constraint tangent A2 L8
  constraint perpendicular L2 L8
  constraint coincident A2 L9.start
  constraint coincident L2 L9.end
  constraint tangent A2 L9
  constraint perpendicular L2 L9
  constraint coincident A1 L10.start
  constraint coincident L0 L10.end
  constraint tangent A1 L10
  constraint perpendicular L0 L10
  constraint coincident A1 L11.start
  constraint coincident L0 L11.end
  constraint tangent A1 L11
  constraint perpendicular L0 L11
  constraint concentric A2 A5
  constraint concentric A4 A6
  constraint concentric A3 A7
  constraint concentric A1 A8
  measures "d298" diameter of A1
  measures "d299" diameter of A2
  measures "d300" distance of L0 A1.centre
  measures "d301" distance of L2 A2.centre
  measures "d302" diameter of A3
  measures "d303" diameter of A4
  measures "d304" distance of L0 A3.centre
  measures "d305" distance of L1 A3.centre
  measures "d306" distance of L2 A4.centre
  measures "d307" distance of L1 A4.centre
  measures "d308" diameter of A5
  measures "d309" diameter of A6
  measures "d310" diameter of A7
  measures "d311" diameter of A8
extrude "Extrude5''" cut sketch "Sketch5" against normal blind 5 contours A5 | A6 | A7 | A8 bodies 6 in component "Lid"
sketch "Sketch8" plane through (0, 83, 0) normal (0, 1, 0) x (-1, 0, 0) in component "Box"
  line L0 (60, -95) -> (-60, -95)
  line L1 (-60, -95) -> (-60, 75)
  line L2 (-60, 75) -> (60, 75)
  line L3 (60, 75) -> (60, -95)
  line L4 (-63, -98) -> (63, -98)
  line L5 (63, -98) -> (63, 78)
  line L6 (63, 78) -> (-63, 78)
  line L7 (-63, 78) -> (-63, -98)
  circle A0 centre (58.5, 0) radius 1.05
  circle A1 centre (-58.5, 0) radius 1.05
  circle A2 centre (58.5, 73.5) radius 1.05
  circle A3 centre (-58.5, 73.5) radius 1.05
  line L8 (-60, 75) -> (-60, -95)
  line L9 (60, 75) -> (-60, 75)
  line L10 (60, -95) -> (60, 75)
  circle A4 centre (-58.5, 0) radius 2.5
  circle A5 centre (-58.5, 73.5) radius 2.5
  circle A6 centre (58.5, 73.5) radius 2.5
  circle A7 centre (58.5, 0) radius 2.5
  line L11 (58.5, 71) -> (60, 71)
  line L12 (56, 73.5) -> (56, 75)
  line L13 (-56, 73.5) -> (-56, 75)
  line L14 (-58.5, 71) -> (-60, 71)
  line L15 (-58.5, 2.5) -> (-60, 2.5)
  line L16 (-58.5, -2.5) -> (-60, -2.5)
  line L17 (58.5, -2.5) -> (60, -2.5)
  line L18 (58.5, 2.5) -> (60, 2.5)
  dimension "d281" = 2.1
  dimension "d282" = 2.1
  dimension "d283" = 2.1
  dimension "d284" = 2.1
  dimension "d286" = 1.5
  dimension "d287" = 1.5
  dimension "d288" = 1.5
  dimension "d289" = 1.5
  dimension "d290" = 1.5
  dimension "d291" = 1.5
  dimension "d292" = 5
  dimension "d293" = 5
  dimension "d294" = 5
  dimension "d295" = 5
  constraint concentric A1 A4
  constraint concentric A3 A5
  constraint concentric A2 A6
  constraint concentric A0 A7
  constraint coincident A6 L11.start
  constraint coincident L3 L11.end
  constraint tangent A6 L11
  constraint perpendicular L3 L11
  constraint coincident A6 L12.start
  constraint coincident L2 L12.end
  constraint tangent A6 L12
  constraint perpendicular L2 L12
  constraint coincident A5 L13.start
  constraint coincident L2 L13.end
  constraint tangent A5 L13
  constraint perpendicular L2 L13
  constraint coincident A5 L14.start
  constraint coincident L8 L14.end
  constraint tangent A5 L14
  constraint perpendicular L8 L14
  constraint coincident A4 L15.start
  constraint coincident L8 L15.end
  constraint tangent A4 L15
  constraint perpendicular L8 L15
  constraint coincident A4 L16.start
  constraint coincident L8 L16.end
  constraint tangent A4 L16
  constraint perpendicular L8 L16
  constraint coincident A7 L17.start
  constraint coincident L3 L17.end
  constraint tangent A7 L17
  constraint perpendicular L3 L17
  constraint coincident A7 L18.start
  constraint coincident L10 L18.end
  constraint tangent A7 L18
  constraint perpendicular L10 L18
  measures "d281" diameter of A0
  measures "d282" diameter of A1
  measures "d283" diameter of A2
  measures "d284" diameter of A3
  measures "d286" distance of A3.centre L8
  measures "d287" distance of A3.centre L9
  measures "d288" distance of A2.centre L10
  measures "d289" distance of A2.centre L9
  measures "d290" distance of A0.centre L10
  measures "d291" distance of A1.centre L8
  measures "d292" diameter of A4
  measures "d293" diameter of A5
  measures "d294" diameter of A6
  measures "d295" diameter of A7
extrude "Extrude12" add sketch "Sketch8" against normal blind 5 contours L3 L10 A7 L17 | L1 L8 A4 L16 | L3 L10 A7 | L1 L8 A4 | L3 L10 A7 L18 | L1 L8 A4 L15 | L3 L10 A6 L11 | L1 L8 A5 L14 | L2 L3 L9 L10 A6 | L1 L2 L8 L9 A5 | L2 L9 A6 L12 | L2 L9 A5 L13 picked at (59.85, 0) picked at (-59.85, 0) picked at (58.3072, 74.849) picked at (-58.3595, 74.849) bodies 1 in component "Box"
sketch "Sketch6" plane through (0, 86, 0) normal (0, 1, 0) x (-1, 0, 0) in component "Lid"
  circle A0 centre (-58.5, 73.5) radius 1.05
  circle A1 centre (-58.5, 0) radius 1.05
  circle A2 centre (58.5, 73.5) radius 1.05
  circle A3 centre (58.5, 0) radius 1.05
  circle A4 centre (0, 0) radius 3.1
  line L0 (63, -10) -> (63, 78)
  line L1 (63, 78) -> (-63, 78)
  line L2 (-63, 78) -> (-63, -10)
  line L3 (-63, -10) -> (63, -10)
  circle A5 centre (-58.5, 0) radius 3
  circle A6 centre (-58.5, 73.5) radius 3
  circle A7 centre (58.5, 73.5) radius 3
  circle A8 centre (58.5, 0) radius 3
  dimension "d314" = 6
  dimension "d315" = 6
  dimension "d316" = 6
  dimension "d317" = 6
  constraint concentric A1 A5
  constraint concentric A0 A6
  constraint concentric A2 A7
  constraint concentric A3 A8
  measures "d314" diameter of A5
  measures "d315" diameter of A6
  measures "d316" diameter of A7
  measures "d317" diameter of A8
extrude "Extrude6" cut sketch "Sketch6" against normal blind 1 contours A5 | A6 | A7 | A8 bodies 6 in component "Lid"
sketch "Sketch7 (2)" plane through (0, 83, 0) normal (0, 1, 0) x (-1, 0, 0) in component "Lid"
  circle A0 centre (-58.5, 0) radius 1.05
  circle A1 centre (58.5, 0) radius 1.05
  circle A2 centre (-58.5, 73.5) radius 1.05
  circle A3 centre (58.5, 73.5) radius 1.05
  line L0 (60, -95) -> (-60, -95)
  line L1 (-60, -95) -> (-60, -2.5)
  line L2 (-60, -2.5) -> (-58.5, -2.5)
  arc A4 (-58.5, -2.5) -> (-58.5, 2.5) centre (-58.5, 0) ccw
  line L3 (-58.5, 2.5) -> (-60, 2.5)
  line L4 (-60, 2.5) -> (-60, 71)
  line L5 (-60, 71) -> (-58.5, 71)
  arc A5 (-58.5, 71) -> (-56, 73.5) centre (-58.5, 73.5) ccw
  line L6 (-56, 73.5) -> (-56, 75)
  line L7 (-56, 75) -> (56, 75)
  line L8 (56, 75) -> (56, 73.5)
  arc A6 (56, 73.5) -> (58.5, 71) centre (58.5, 73.5) ccw
  line L9 (58.5, 71) -> (60, 71)
  line L10 (60, 71) -> (60, 2.5)
  line L11 (60, 2.5) -> (58.5, 2.5)
  arc A7 (58.5, 2.5) -> (58.5, -2.5) centre (58.5, 0) ccw
  line L12 (58.5, -2.5) -> (60, -2.5)
  line L13 (60, -2.5) -> (60, -95)
  line L14 (-63, -98) -> (63, -98)
  line L15 (63, -98) -> (63, 78)
  line L16 (63, 78) -> (-63, 78)
  line L17 (-63, 78) -> (-63, -98)
  line L18 (63, -98) -> (-63, -98)
  line L19 (-63, -98) -> (-63, -11)
  line L20 (-63, -11) -> (63, -11)
  line L21 (63, -11) -> (63, -98)
  dimension "d320" = 126
  dimension "d321" = 87
  constraint horizontal L18
  constraint vertical L19
  constraint horizontal L20
  constraint vertical L21
  constraint coincident L14.end L15.start
  measures "d320" distance of L14.end L14.start
  measures "d321" distance of L14.end L20.end
extrude "Extrude7" add sketch "Sketch7 (2)" along normal blind 3 separate body contours L0 L1 L13 L14 L15 L17 L18 L19 L20 L21 | L0 L1 L13 L20 makes body 7 in component "Lid"
ref_plane "WorkPlane1" through (63, 0, 0) normal (1, 0, 0) x (0, 1, 0) in component "Box"
sketch "Sketch9" plane through (63, 0, 0) normal (1, 0, 0) x (0, 0, -1) in component "Box"
  line L0 (98, 83) -> (101.5, 83) construction
  circle A0 centre (101.5, 83) radius 3.5
  circle A1 centre (101.5, 83) radius 1.5
  line L1 (104.2361, 80.8174) -> (98, 73)
  line L2 (98, 73) -> (98, 83)
  dimension "d329" = 3.5
  dimension "d330" = 7
  dimension "d331" = 3
  constraint horizontal L0
  constraint coincident L0.end A0.centre
  constraint coincident A0 L1.start
  constraint tangent A0 L1
  constraint tangent A0 L2
  measures "d329" distance of L0.start L0.end
  measures "d330" diameter of A0
  measures "d331" diameter of A1
extrude "Extrude13" add sketch "Sketch9" against normal blind 8 from surface at -21 bodies 1 in component "Box"
pattern_linear "R-Pattern1" count 2 spacing 16.5 along (-1, 0, 0) of "Extrude13" in component "Box"
pattern_linear "R-Pattern2" count 2 spacing 59.5 along (-1, 0, 0) of "Extrude13", "R-Pattern1" in component "Box"
sketch "Sketch8 (2)" plane through (63, 0, 0) normal (1, 0, 0) x (0, 0, -1) in component "Lid"
  line L0 (11, 83) -> (98, 83)
  line L1 (98, 83) -> (98, 86)
  line L2 (98, 86) -> (11, 86)
  line L3 (11, 86) -> (11, 83)
  line L4 (97.5, 86) -> (97.5, 83)
  dimension "d343" = 3
  dimension "d344" = 0.5
  constraint coincident L2 L4.start
  constraint perpendicular L2 L4
  measures "d343" distance of L4.start L4.end
  measures "d344" distance of L1 L4
extrude "Extrude8" cut sketch "Sketch8 (2)" against normal blind 8.2 from surface at -20.9 contours L0 L1 L2 L4 bodies 7 in component "Lid"
pattern_linear "R-Pattern1'" count 2 spacing 16.5 along (-1, 0, 0) of "Extrude8" in component "Lid"
pattern_linear "R-Pattern2'" count 2 spacing 59.5 along (-1, 0, 0) of "Extrude8", "R-Pattern1'" in component "Lid"
sketch "Sketch9 (2)" plane through (33.9, 0, 0) normal (1, 0, 0) x (0, 0, -1) in component "Lid"
  line L0 (97.5, 86) -> (97.5, 83)
  line L1 (97.5, 83) -> (98, 83)
  line L2 (98, 83) -> (98, 86)
  line L3 (98, 86) -> (97.5, 86)
  circle A0 centre (101.5, 83) radius 1.5
  circle A1 centre (101.5, 83) radius 3.5
  line L4 (101.5, 86.5) -> (98, 86)
  dimension "d356" = 3
  dimension "d357" = 7
  constraint concentric A0 A1
  constraint coincident A1 L4.start
  constraint coincident L2.end L3.start
  measures "d356" diameter of A0
  measures "d357" diameter of A1
extrude "Extrude9'" add sketch "Sketch9 (2)" against normal up to surface (8.3 mm away) contours L2 A1 L4 | A1 L4 | A0 picked at (101.136, 85.7853) bodies 7 in component "Lid"
pattern_linear "R-Pattern3" count 2 spacing 59.5 along (-1, 0, 0) of "Extrude9'" in component "Lid"
sketch "Sketch10" plane through (33.9, 0, 0) normal (1, 0, 0) x (0, 0, -1) in component "Lid"
  line L0 (97.5, 86) -> (97.5, 83)
  line L1 (97.5, 83) -> (98, 83)
  arc A0 (98, 83) -> (101.5, 86.5) centre (101.5, 83) ccw
  line L2 (101.5, 86.5) -> (98, 86)
  line L3 (98, 86) -> (97.5, 86)
  circle A1 centre (101.5, 83) radius 1.5
  dimension "d364" = 3
  constraint concentric A0 A1
  measures "d364" diameter of A1
extrude "Extrude10'" cut sketch "Sketch10" against normal up to surface (67.8 mm away) contours A1 bodies 7 in component "Lid"
sketch "Sketch1 (6)" plane through (42, 0, 0) normal (1, 0, 0) x (0, 0, -1) in component "Hinge_pipe"
  circle A0 centre (101.5, 83) radius 1.5
  arc A1 (104.2361, 80.8174) -> (98, 83) centre (101.5, 83) ccw
  line L0 (98, 83) -> (98, 73)
  line L1 (98, 73) -> (104.2361, 80.8174)
  circle A2 centre (101.5, 83) radius 1.4
  dimension "d367" = 2.8
  constraint concentric A0 A2
  measures "d367" diameter of A2
extrude "Extrude1'''''" add sketch "Sketch1 (6)" against normal blind 87 separate body contours A2 makes body 8 in component "Hinge_pipe"
sketch "Sketch2 (6)" plane through (42, 0, 0) normal (1, 0, 0) x (0, 0, -1) in component "Hinge_pipe"
  circle A0 centre (101.5, 83) radius 1.4
  circle A1 centre (101.5, 83) radius 2.5
  dimension "d370" = 5
  constraint concentric A0 A1
  measures "d370" diameter of A1
extrude "Extrude2'''''" add sketch "Sketch2 (6)" along normal blind 2 contours A0 | A1 bodies 8 in component "Hinge_pipe"
sketch "Sketch2 (7)" plane through (-45, 0, 0) normal (-1, 0, 0) x (0, 0, 1) in component "Pipe_end"
  circle A0 centre (-101.5, 83) radius 1.4
  circle A1 centre (-101.5, 83) radius 1.45
  circle A2 centre (-101.5, 83) radius 2
  dimension "d373" = 2.9
  dimension "d374" = 4
  constraint concentric A0 A1
  constraint concentric A1 A2
  measures "d373" diameter of A1
  measures "d374" diameter of A2
sketch "Sketch3 (4)" plane through (-46, 0, 0) normal (-1, 0, 0) x (0, 0, 1) in component "Pipe_end"
  circle A0 centre (-101.5, 83) radius 1.45
  circle A1 centre (-101.5, 83) radius 2
  circle A2 centre (-101.5, 83) radius 2
  dimension "d377" = 4
  constraint concentric A0 A2
  measures "d377" diameter of A2
sketch "Sketch4 (2)" plane through (-45, 0, 0) normal (-1, 0, 0) x (0, 0, 1) in component "Pipe_end"
  circle A0 centre (-101.5, 83) radius 1.4
  circle A1 centre (-101.5, 83) radius 2.5
  circle A2 centre (-101.5, 83) radius 1.45
  dimension "d380" = 5
  dimension "d381" = 2.9
  constraint concentric A0 A1
  constraint concentric A1 A2
  measures "d380" diameter of A1
  measures "d381" diameter of A2
extrude "Extrude3''''" add sketch "Sketch4 (2)" along normal blind 2 and the other way blind 2 separate body contours A1 makes body 9 in component "Pipe_end"
sketch "Sketch5 (2)" plane through (-47, 0, 0) normal (-1, 0, 0) x (0, 0, 1) in component "Pipe_end"
  circle A0 centre (-101.5, 83) radius 1.45
  circle A1 centre (-101.5, 83) radius 2.5
extrude "Extrude4''''" add sketch "Sketch5 (2)" along normal blind 2 contours A0 | A1 bodies 9 in component "Pipe_end"